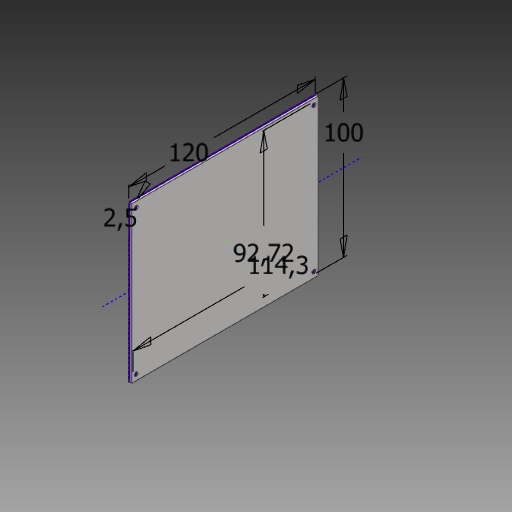
# Autodesk Inventor part: MotorController
Saved by Autodesk Inventor 2019.1 (Build 231200000, 200)
## iProperties
Created: 2018-09-15
Part Number: MotorController
Material: Generisch
Document SubType Name: Modeling
Designer: JochenAlt
Density: 1 g/cm^3
Appearance: Vorgabe
Author: JochenAlt
Autodesk Inventor part; units mm, degrees
ref_plane "YZ Plane" through (0, 0, 0) normal (1, 0, 0) x (0, 1, 0)
ref_plane "XZ Plane" through (0, 0, 0) normal (0, 1, 0) x (-1, 0, 0)
ref_plane "XY Plane" through (0, 0, 0) normal (0, 0, 1) x (1, 0, 0)
sketch "Skizze1" plane through (0, 0, 0) normal (1, 0, 0) x (0, 1, 0)
  line L0 (-60, 50) -> (60, 50)
  line L1 (60, 50) -> (60, -50)
  line L2 (60, -50) -> (-60, -50)
  line L3 (-60, -50) -> (-60, 50)
  line L4 (0, 37.4988) -> (0, -37.4988) construction
  line L5 (-78.3748, 0) -> (89.6252, 0) construction
  line L6 (-57.15, 46.36) -> (57.15, 46.36) construction
  line L7 (57.15, 46.36) -> (57.15, -46.36) construction
  line L8 (57.15, -46.36) -> (-57.15, -46.36) construction
  line L9 (-57.15, -46.36) -> (-57.15, 46.36) construction
  circle A0 centre (-57.15, 46.36) radius 1.25
  circle A1 centre (57.15, 46.36) radius 1.25
  circle A2 centre (-57.15, -46.36) radius 1.25
  circle A3 centre (57.15, -46.36) radius 1.25
  line L10 (-60, 50) -> (60.1722, 49.7926) construction
  line L11 (60.1722, 49.7926) -> (60, -50) construction
  line L12 (60, -50) -> (-60.1722, -49.7926) construction
  line L13 (-60.1722, -49.7926) -> (-60, 50) construction
  point P0 (0, 0)
  point P1 (0, 0)
  point P2 (0, 0)
  dimension "d0" = 120
  dimension "d1" = 100
  dimension "d4" = 2.5
  dimension "d5" = 114.3
  dimension "d6" = 92.72
  constraints: 20 end point, 5 coincident, 4 centre point, 4 parallel, 3 equal radius, 2 horizontal, 2 midpoint, 2 perpendicular, 2 point on line, 6 other
  measures "d0" distance of L0.start L0.end
  measures "d1" distance of L0.end L1.end
  measures "d4" diameter of A0
  measures "d5" distance of L7.end L8.end
  measures "d6" distance of L6.end L7.end
extrude "Extrusion1" add sketch "Skizze1" along normal blind 2
